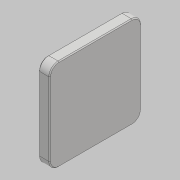
# Autodesk Inventor part: exercise3-6
Saved by Autodesk Inventor 2018 (Build 220112000, 112)
## iProperties
Created: 2020-09-23
Part Number: exercise3-6
Material: 一般
Document SubType Name: Modeling
Designer: 王鼎鈞
Density: 1 g/cm^3
Appearance: 預設
Author: 王鼎鈞
Autodesk Inventor part; units mm, degrees
ref_plane "YZ Plane" through (0, 0, 0) normal (1, 0, 0) x (0, 1, 0)
ref_plane "XZ Plane" through (0, 0, 0) normal (0, 1, 0) x (-1, 0, 0)
ref_plane "XY Plane" through (0, 0, 0) normal (0, 0, 1) x (1, 0, 0)
sketch "草圖1" plane through (0, 0, 0) normal (1, 0, 0) x (0, 1, 0)
  line L0 (-50, 50) -> (50, 50)
  line L1 (50, 50) -> (50, -50)
  line L2 (50, -50) -> (-50, -50)
  line L3 (-50, -50) -> (-50, 50)
  line L4 (-50, 50) -> (50, -50) construction
  line L5 (50, 50) -> (-50, -50) construction
  point P0 (0, 0)
  dimension "d0" = 100
  dimension "d1" = 100
  constraints: 12 end point, 2 midpoint, 2 parallel, 1 horizontal, 1 perpendicular
  measures "d0" distance of L1.end L2.end
  measures "d1" distance of L2.end L0.start
extrude "擠出1" add sketch "草圖1" along normal blind 12
fillet "圓角1" radius 10 4 edges at (6, 50, 50) (6, 50, -50) (6, -50, 50) (6, -50, -50)
chamfer "倒角1" distance 1 angle 45 16 edges at (12, 0, 50) (12, -47.0711, 47.0711) (12, -50, 0) (12, -47.0711, -47.0711) (12, 0, -50) (12, 47.0711, -47.0711) (12, 50, 0) (12, 47.0711, 47.0711) (0, 0, 50) (0, 47.0711, 47.0711) (0, 50, 0) (0, 47.0711, -47.0711) (0, 0, -50) (0, -47.0711, -47.0711) (0, -50, 0) (0, -47.0711, 47.0711)
